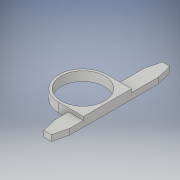
# Autodesk Inventor part: Headbar_D_Shape_unfinished
Saved by Autodesk Inventor 2019 (Build 230136000, 136)
## iProperties
Created: 2019-12-06
Part Number: Headbar_D_Shape_unfinished
Material: Generic
Document SubType Name: Modeling
Designer: Eivind
Density: 1 g/cm^3
Appearance: Default
Author: Eivind
Autodesk Inventor part; units mm, degrees
ref_plane "YZ Plane" through (0, 0, 0) normal (1, 0, 0) x (0, 1, 0)
ref_plane "XZ Plane" through (0, 0, 0) normal (0, 1, 0) x (-1, 0, 0)
ref_plane "XY Plane" through (0, 0, 0) normal (0, 0, 1) x (1, 0, 0)
sketch "Sketch1" plane through (0, 0, 0) normal (0, 1, 0) x (-1, 0, 0)
  line L0 (0.8, 12.8) -> (-0.8, 12.8)
  line L1 (-1.6, 9.6) -> (-1.6, -9.6)
  line L2 (-0.8, -12.8) -> (0.8, -12.8)
  line L3 (1.6, -9.6) -> (1.6, 9.6)
  line L4 (1.6, 9.6) -> (0.8, 12.8)
  line L5 (-1.6, 9.6) -> (-0.8, 12.8)
  line L6 (1.6, -9.6) -> (0.8, -12.8)
  line L7 (-1.6, -9.6) -> (-0.8, -12.8)
  line L8 (-1.6, 6.2) -> (-1.6, -4.2)
  point P0 (0, 0)
  point P1 (1.6, 12.8)
  point P2 (-1.6, 12.8)
  point P3 (1.6, -12.8)
  dimension "d0" = 25.6
  dimension "d1" = 3.2
  dimension "d2" = 1.6
  dimension "d3" = 12.8
  dimension "d4" = 3.2
  dimension "d12" = 0
  constraints: 18 end point, 6 point on line, 2 parallel, 1 horizontal, 1 perpendicular
  measures "d0" distance of point (1.6, -12.8) point (1.6, 12.8)
  measures "d1" distance of point (1.6, 12.8) point (-1.6, 12.8)
  measures "d2" distance from line of L1 point (0, 0)
  measures "d3" distance from line of L2 point (0, 0)
  measures "d4" distance from line of L3.end L0
  measures "d12" distance between parallel lines of L1 L8
extrude "Extrusion1" add sketch "Sketch1" along normal blind 1.27
sketch "Sketch4" plane through (0, 0, 0) normal (0, -1, 0) x (1, 0, 0)
  line L0 (1.6, -3.7217) -> (-3.7, -3.7217)
  line L1 (-3.7, 6.6783) -> (1.6, 6.6783)
  line L2 (1.6, 6.6783) -> (1.6, -3.7217)
  line L3 (1.6, 9.6) -> (1.6, -9.6) projected
  arc A0 (-3.7, 6.6783) -> (-3.7, -3.7217) centre (-3.7, 1.4783) ccw
  point P0 (0, 0)
  dimension "d23" = 10.4
  dimension "d24" = 0
  dimension "d27" = 5.3
  constraints: 6 end point, 2 point on circle, 1 centre point, 1 horizontal, 1 parallel
  measures "d23" distance between parallel lines of L0 L1
  measures "d24" distance between parallel lines of L3 L2
  measures "d27" distance from line of L2 A0.centre
extrude "Extrusion2" add sketch "Sketch4" against normal blind 2
sketch "Sketch5" plane through (0, 2, 0) normal (0, 1, 0) x (1, 0, 0)
  circle A0 centre (-3.7, -1.4783) radius 4.7
  line L0 (1.6, -6.6783) -> (1.6, 3.7217) projected
  line L1 (-3.7, -6.6783) -> (1.6, -6.6783) projected
  point P0 (0, 0)
  dimension "d30" = 9.4
  dimension "d31" = 5.3
  dimension "d32" = 5.2
  constraints: 1 centre point
  measures "d30" diameter of A0
  measures "d31" distance from line of L0 A0.centre
  measures "d32" distance from line of L1 A0.centre
extrude "Extrusion3" cut sketch "Sketch5" against normal blind 2
body "Solid1"
